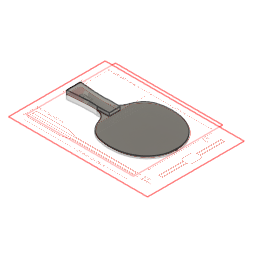
ping pong blade v3 (Autodesk Fusion 360 design; units mm, degrees)
Autodesk Fusion 360 part; units mm, degrees
sketch "Sketch1" plane through (0, 0, 0) normal (0, 0, 1) x (1, 0, 0)
  line L0 (-50.4364, 20) -> (-50.4364, 66.2164)
  line L1 (-50.4364, 20) -> (-50.4364, -26.2164)
  line L2 (-162.6012, 20) -> (-162.6012, 37.8)
  spline S0 degree 5 poles (-162.6012, 37.8) (-162.4087, 37.7675) (-161.9968, 37.7008) (-161.2988, 37.596) (-160.2074, 37.4467) (-158.5833, 37.2448) (-156.7226, 37.0291) (-154.6748, 36.8033) (-152.512, 36.5725) (-150.3117, 36.3424) (-148.1418, 36.1177) (-146.0475, 35.9017) (-144.0316, 35.6944) (-142.0557, 35.4931) (-140.0634, 35.2939) (-137.9994, 35.0931) (-135.8278, 34.8889) (-133.5564, 34.6833) (-131.2346, 34.4817) (-128.928, 34.291) (-126.6995, 34.1181) (-124.5892, 33.968) (-122.5913, 33.8422) (-120.6411, 33.7376) (-118.6447, 33.6482) (-116.5034, 33.5668) (-114.1389, 33.4868) (-111.5213, 33.4035) (-108.6885, 33.3162) (-105.7218, 33.2269) (-102.7286, 33.1405) (-99.8212, 33.0642) (-97.0976, 33.0075) (-94.623, 32.9812) (-92.4049, 32.998) (-90.397, 33.0706) (-88.525, 33.21) (-86.708, 33.4235) (-84.879, 33.7126) (-83.0115, 34.0709) (-81.1155, 34.4864) (-79.2188, 34.9473) (-77.3539, 35.4469) (-75.5416, 35.9885) (-73.7777, 36.5903) (-72.0452, 37.2766) (-70.3251, 38.0715) (-68.6068, 38.9915) (-66.9017, 40.0363) (-65.2418, 41.1906) (-63.6663, 42.433) (-62.2115, 43.7433) (-60.8996, 45.1106) (-59.7266, 46.542) (-58.6672, 48.0584) (-57.6848, 49.6888) (-56.7383, 51.464) (-55.792, 53.4107) (-54.8211, 55.5471) (-53.8091, 57.8853) (-52.7461, 60.4323) (-51.8509, 62.6395) (-51.1537, 64.3907) (-50.6774, 65.6008) (-50.4364, 66.2164) knots 0 0 0 0 0 0 0.01666667 0.03333333 0.05 0.06666667 0.08333333 0.1 0.11666667 0.13333333 0.15 0.16666667 0.18333333 0.2 0.21666667 0.23333333 0.25 0.26666667 0.28333333 0.3 0.31666667 0.33333333 0.35 0.36666667 0.38333333 0.4 0.41666667 0.43333333 0.45 0.46666667 0.48333333 0.5 0.51666667 0.53333333 0.55 0.56666667 0.58333333 0.6 0.61666667 0.63333333 0.65 0.66666667 0.68333333 0.7 0.71666667 0.73333333 0.75 0.76666667 0.78333333 0.8 0.81666667 0.83333333 0.85 0.86666667 0.88333333 0.9 0.91666667 0.93333333 0.95 0.96666667 0.98333333 1 1 1 1 1 1
  spline S1 degree 5 poles (-50.4364, 66.2164) (-50.3519, 66.4112) (-50.1757, 66.8083) (-49.8889, 67.4271) (-49.4619, 68.2982) (-48.8547, 69.4625) (-48.1772, 70.6978) (-47.4359, 71.9953) (-46.6416, 73.3403) (-45.8078, 74.7134) (-44.9479, 76.0937) (-44.072, 77.4613) (-43.185, 78.7999) (-42.2827, 80.0994) (-41.3532, 81.3565) (-40.382, 82.5722) (-39.3568, 83.7496) (-38.2715, 84.8926) (-37.1319, 86.0029) (-35.9566, 87.0799) (-34.7693, 88.121) (-33.5926, 89.1233) (-32.4408, 90.0841) (-31.3134, 91.0023) (-30.1901, 91.8786) (-29.0408, 92.7154) (-27.8344, 93.5153) (-26.5475, 94.2804) (-25.1741, 95.0118) (-23.7297, 95.7088) (-22.2422, 96.3696) (-20.7456, 96.9918) (-19.2732, 97.5726) (-17.8503, 98.1091) (-16.4878, 98.5993) (-15.1849, 99.042) (-13.9302, 99.4379) (-12.7036, 99.7901) (-11.4773, 100.1046) (-10.22, 100.3903) (-8.9052, 100.6573) (-7.5176, 100.9156) (-6.0613, 101.1732) (-4.5656, 101.4355) (-3.0718, 101.7048) (-1.6195, 101.9808) (-0.2335, 102.2603) (1.0906, 102.538) (2.3958, 102.806) (3.7421, 103.0559) (5.1885, 103.2799) (6.7748, 103.4722) (8.4989, 103.6309) (10.315, 103.7579) (12.155, 103.8571) (13.9436, 103.9335) (15.617, 103.9914) (17.138, 104.0331) (18.5172, 104.0573) (19.8025, 104.0605) (21.056, 104.0389) (22.3366, 103.9907) (23.6775, 103.9184) (25.0748, 103.8296) (26.5038, 103.7337) (27.9321, 103.6387) (29.332, 103.5492) (30.6963, 103.4618) (32.0362, 103.3676) (33.3674, 103.2568) (34.7009, 103.1228) (36.0308, 102.9669) (37.3268, 102.8014) (38.555, 102.6418) (39.6952, 102.5008) (40.7596, 102.3813) (41.8115, 102.2697) (42.9331, 102.1439) (44.1925, 101.9806) (45.6078, 101.7646) (47.1227, 101.4944) (48.6444, 101.1781) (50.0749, 100.8298) (51.3416, 100.4659) (52.4354, 100.1015) (53.4214, 99.7468) (54.3927, 99.4068) (55.4411, 99.0795) (56.6121, 98.7537) (57.9048, 98.4117) (59.2923, 98.0347) (60.7347, 97.6062) (62.1975, 97.1178) (63.6625, 96.5716) (65.1218, 95.9761) (66.575, 95.3435) (68.0244, 94.6863) (69.4712, 94.0139) (70.9122, 93.3296) (72.341, 92.6324) (73.7506, 91.9192) (75.1345, 91.1862) (76.489, 90.4307) (77.8147, 89.6534) (79.1164, 88.8568) (80.4014, 88.0438) (81.6783, 87.2155) (82.9563, 86.37) (84.2434, 85.4998) (85.546, 84.5942) (86.8673, 83.6418) (88.2065, 82.6336) (89.5581, 81.566) (90.91, 80.4435) (92.2446, 79.28) (93.5423, 78.0932) (94.7848, 76.902) (95.958, 75.7222) (97.0558, 74.5632) (98.0833, 73.4234) (99.0553, 72.2922) (99.9911, 71.1542) (100.9108, 69.9933) (101.8313, 68.7959) (102.7615, 67.5557) (103.7029, 66.273) (104.6516, 64.9514) (105.6008, 63.5956) (106.5423, 62.2091) (107.4689, 60.7914) (108.3755, 59.3369) (109.2582, 57.8381) (110.1142, 56.287) (110.941, 54.6779) (111.7362, 53.0089) (112.4967, 51.2846) (113.2191, 49.5157) (113.8998, 47.7159) (114.5354, 45.9004) (115.123, 44.083) (115.6604, 42.275) (116.1465, 40.4817) (116.5815, 38.702) (116.9663, 36.9306) (117.3026, 35.159) (117.5921, 33.377) (117.8368, 31.5747) (118.0382, 29.7435) (118.1974, 27.8777) (118.3152, 25.9734) (118.3921, 24.028) (118.4211, 22.4381) (118.4245, 21.2265) (118.4186, 20.4102) (118.4136, 20) knots 0 0 0 0 0 0 0.00666667 0.01333333 0.02 0.02666667 0.03333333 0.04 0.04666667 0.05333333 0.06 0.06666667 0.07333333 0.08 0.08666667 0.09333333 0.1 0.10666667 0.11333333 0.12 0.12666667 0.13333333 0.14 0.14666667 0.15333333 0.16 0.16666667 0.17333333 0.18 0.18666667 0.19333333 0.2 0.20666667 0.21333333 0.22 0.22666667 0.23333333 0.24 0.24666667 0.25333333 0.26 0.26666667 0.27333333 0.28 0.28666667 0.29333333 0.3 0.30666667 0.31333333 0.32 0.32666667 0.33333333 0.34 0.34666667 0.35333333 0.36 0.36666667 0.37333333 0.38 0.38666667 0.39333333 0.4 0.40666667 0.41333333 0.42 0.42666667 0.43333333 0.44 0.44666667 0.45333333 0.46 0.46666667 0.47333333 0.48 0.48666667 0.49333333 0.5 0.50666667 0.51333333 0.52 0.52666667 0.53333333 0.54 0.54666667 0.55333333 0.56 0.56666667 0.57333333 0.58 0.58666667 0.59333333 0.6 0.60666667 0.61333333 0.62 0.62666667 0.63333333 0.64 0.64666667 0.65333333 0.66 0.66666667 0.67333333 0.68 0.68666667 0.69333333 0.7 0.70666667 0.71333333 0.72 0.72666667 0.73333333 0.74 0.74666667 0.75333333 0.76 0.76666667 0.77333333 0.78 0.78666667 0.79333333 0.8 0.80666667 0.81333333 0.82 0.82666667 0.83333333 0.84 0.84666667 0.85333333 0.86 0.86666667 0.87333333 0.88 0.88666667 0.89333333 0.9 0.90666667 0.91333333 0.92 0.92666667 0.93333333 0.94 0.94666667 0.95333333 0.96 0.96666667 0.97333333 0.98 0.98666667 0.99333333 1 1 1 1 1 1
  line L3 (-50.4364, 18.5) -> (-162.6012, 18.5) construction
  line L4 (-50.4364, 18.5) -> (130, 18.5) construction
  spline S2 degree 5 poles (118.4136, 20) (118.4136, 19.94) (118.4136, 19.82) (118.4136, 19.64) (118.4136, 19.4) (118.4136, 19.1) (118.4136, 18.86) (118.4136, 18.68) (118.4136, 18.56) (118.4136, 18.5) knots 0 0 0 0 0 0 0.2 0.4 0.6 0.8 1 1 1 1 1 1
  line L5 (-162.6012, 18.5) -> (-162.6012, 20)
  spline S3 degree 5 poles (118.4136, 17) (118.4136, 17.06) (118.4136, 17.18) (118.4136, 17.36) (118.4136, 17.6) (118.4136, 17.9) (118.4136, 18.14) (118.4136, 18.32) (118.4136, 18.44) (118.4136, 18.5) knots 0 0 0 0 0 0 0.2 0.4 0.6 0.8 1 1 1 1 1 1
  line L6 (118.4136, 20.153) -> (118.4136, 19.847)
  line L7 (118.4136, 18.653) -> (118.4136, 18.347)
  line L8 (118.4136, 16.847) -> (118.4136, 17.153)
  line L9 (118.4136, 18.347) -> (118.4136, 18.653)
  spline S4 degree 5 poles (-162.6012, -0.8) (-162.4087, -0.7675) (-161.9968, -0.7008) (-161.2988, -0.596) (-160.2074, -0.4467) (-158.5833, -0.2448) (-156.7226, -0.0291) (-154.6748, 0.1967) (-152.512, 0.4275) (-150.3117, 0.6576) (-148.1418, 0.8823) (-146.0475, 1.0983) (-144.0316, 1.3056) (-142.0557, 1.5069) (-140.0634, 1.7061) (-137.9994, 1.9069) (-135.8278, 2.1111) (-133.5564, 2.3167) (-131.2346, 2.5183) (-128.928, 2.709) (-126.6995, 2.8819) (-124.5892, 3.032) (-122.5913, 3.1578) (-120.6411, 3.2624) (-118.6447, 3.3518) (-116.5034, 3.4332) (-114.1389, 3.5132) (-111.5213, 3.5965) (-108.6885, 3.6838) (-105.7218, 3.7731) (-102.7286, 3.8595) (-99.8212, 3.9358) (-97.0976, 3.9925) (-94.623, 4.0188) (-92.4049, 4.002) (-90.397, 3.9294) (-88.525, 3.79) (-86.708, 3.5765) (-84.879, 3.2874) (-83.0115, 2.9291) (-81.1155, 2.5136) (-79.2188, 2.0527) (-77.3539, 1.5531) (-75.5416, 1.0115) (-73.7777, 0.4097) (-72.0452, -0.2766) (-70.3251, -1.0715) (-68.6068, -1.9915) (-66.9017, -3.0363) (-65.2418, -4.1906) (-63.6663, -5.433) (-62.2115, -6.7433) (-60.8996, -8.1106) (-59.7266, -9.542) (-58.6672, -11.0584) (-57.6848, -12.6888) (-56.7383, -14.464) (-55.792, -16.4107) (-54.8211, -18.5471) (-53.8091, -20.8853) (-52.7461, -23.4323) (-51.8509, -25.6395) (-51.1537, -27.3907) (-50.6774, -28.6008) (-50.4364, -29.2164) knots 0 0 0 0 0 0 0.01666667 0.03333333 0.05 0.06666667 0.08333333 0.1 0.11666667 0.13333333 0.15 0.16666667 0.18333333 0.2 0.21666667 0.23333333 0.25 0.26666667 0.28333333 0.3 0.31666667 0.33333333 0.35 0.36666667 0.38333333 0.4 0.41666667 0.43333333 0.45 0.46666667 0.48333333 0.5 0.51666667 0.53333333 0.55 0.56666667 0.58333333 0.6 0.61666667 0.63333333 0.65 0.66666667 0.68333333 0.7 0.71666667 0.73333333 0.75 0.76666667 0.78333333 0.8 0.81666667 0.83333333 0.85 0.86666667 0.88333333 0.9 0.91666667 0.93333333 0.95 0.96666667 0.98333333 1 1 1 1 1 1
  line L10 (-171.3092, 39.2715) -> (-153.8933, 36.3285)
  line L11 (-56.351, 51.1084) -> (-44.5217, 81.3245)
  line L12 (-171.3092, -2.2715) -> (-153.8933, 0.6715)
  line L13 (-56.351, -14.1084) -> (-44.5217, -44.3245)
  spline S5 degree 5 poles (-50.4364, -29.2164) (-50.3519, -29.4112) (-50.1757, -29.8083) (-49.8889, -30.4271) (-49.4619, -31.2982) (-48.8547, -32.4625) (-48.1772, -33.6978) (-47.4359, -34.9953) (-46.6416, -36.3403) (-45.8078, -37.7134) (-44.9479, -39.0937) (-44.072, -40.4613) (-43.185, -41.7999) (-42.2827, -43.0994) (-41.3532, -44.3565) (-40.382, -45.5722) (-39.3568, -46.7496) (-38.2715, -47.8926) (-37.1319, -49.0029) (-35.9566, -50.0799) (-34.7693, -51.121) (-33.5926, -52.1233) (-32.4408, -53.0841) (-31.3134, -54.0023) (-30.1901, -54.8786) (-29.0408, -55.7154) (-27.8344, -56.5153) (-26.5475, -57.2804) (-25.1741, -58.0118) (-23.7297, -58.7088) (-22.2422, -59.3696) (-20.7456, -59.9918) (-19.2732, -60.5726) (-17.8503, -61.1091) (-16.4878, -61.5993) (-15.1849, -62.042) (-13.9302, -62.4379) (-12.7036, -62.7901) (-11.4773, -63.1046) (-10.22, -63.3903) (-8.9052, -63.6573) (-7.5176, -63.9156) (-6.0613, -64.1732) (-4.5656, -64.4355) (-3.0718, -64.7048) (-1.6195, -64.9808) (-0.2335, -65.2603) (1.0906, -65.538) (2.3958, -65.806) (3.7421, -66.0559) (5.1885, -66.2799) (6.7748, -66.4722) (8.4989, -66.6309) (10.315, -66.7579) (12.155, -66.8571) (13.9436, -66.9335) (15.617, -66.9914) (17.138, -67.0331) (18.5172, -67.0573) (19.8025, -67.0605) (21.056, -67.0389) (22.3366, -66.9907) (23.6775, -66.9184) (25.0748, -66.8296) (26.5038, -66.7337) (27.9321, -66.6387) (29.332, -66.5492) (30.6963, -66.4618) (32.0362, -66.3676) (33.3674, -66.2568) (34.7009, -66.1228) (36.0308, -65.9669) (37.3268, -65.8014) (38.555, -65.6418) (39.6952, -65.5008) (40.7596, -65.3813) (41.8115, -65.2697) (42.9331, -65.1439) (44.1925, -64.9806) (45.6078, -64.7646) (47.1227, -64.4944) (48.6444, -64.1781) (50.0749, -63.8298) (51.3416, -63.4659) (52.4354, -63.1015) (53.4214, -62.7468) (54.3927, -62.4068) (55.4411, -62.0795) (56.6121, -61.7537) (57.9048, -61.4117) (59.2923, -61.0347) (60.7347, -60.6062) (62.1975, -60.1178) (63.6625, -59.5716) (65.1218, -58.9761) (66.575, -58.3435) (68.0244, -57.6863) (69.4712, -57.0139) (70.9122, -56.3296) (72.341, -55.6324) (73.7506, -54.9192) (75.1345, -54.1862) (76.489, -53.4307) (77.8147, -52.6534) (79.1164, -51.8568) (80.4014, -51.0438) (81.6783, -50.2155) (82.9563, -49.37) (84.2434, -48.4998) (85.546, -47.5942) (86.8673, -46.6418) (88.2065, -45.6336) (89.5581, -44.566) (90.91, -43.4435) (92.2446, -42.28) (93.5423, -41.0932) (94.7848, -39.902) (95.958, -38.7222) (97.0558, -37.5632) (98.0833, -36.4234) (99.0553, -35.2922) (99.9911, -34.1542) (100.9108, -32.9933) (101.8313, -31.7959) (102.7615, -30.5557) (103.7029, -29.273) (104.6516, -27.9514) (105.6008, -26.5956) (106.5423, -25.2091) (107.4689, -23.7914) (108.3755, -22.3369) (109.2582, -20.8381) (110.1142, -19.287) (110.941, -17.6779) (111.7362, -16.0089) (112.4967, -14.2846) (113.2191, -12.5157) (113.8998, -10.7159) (114.5354, -8.9004) (115.123, -7.083) (115.6604, -5.275) (116.1465, -3.4817) (116.5815, -1.702) (116.9663, 0.0694) (117.3026, 1.841) (117.5921, 3.623) (117.8368, 5.4253) (118.0382, 7.2565) (118.1974, 9.1223) (118.3152, 11.0266) (118.3921, 12.972) (118.4211, 14.5619) (118.4245, 15.7735) (118.4186, 16.5898) (118.4136, 17) knots 0 0 0 0 0 0 0.00666667 0.01333333 0.02 0.02666667 0.03333333 0.04 0.04666667 0.05333333 0.06 0.06666667 0.07333333 0.08 0.08666667 0.09333333 0.1 0.10666667 0.11333333 0.12 0.12666667 0.13333333 0.14 0.14666667 0.15333333 0.16 0.16666667 0.17333333 0.18 0.18666667 0.19333333 0.2 0.20666667 0.21333333 0.22 0.22666667 0.23333333 0.24 0.24666667 0.25333333 0.26 0.26666667 0.27333333 0.28 0.28666667 0.29333333 0.3 0.30666667 0.31333333 0.32 0.32666667 0.33333333 0.34 0.34666667 0.35333333 0.36 0.36666667 0.37333333 0.38 0.38666667 0.39333333 0.4 0.40666667 0.41333333 0.42 0.42666667 0.43333333 0.44 0.44666667 0.45333333 0.46 0.46666667 0.47333333 0.48 0.48666667 0.49333333 0.5 0.50666667 0.51333333 0.52 0.52666667 0.53333333 0.54 0.54666667 0.55333333 0.56 0.56666667 0.57333333 0.58 0.58666667 0.59333333 0.6 0.60666667 0.61333333 0.62 0.62666667 0.63333333 0.64 0.64666667 0.65333333 0.66 0.66666667 0.67333333 0.68 0.68666667 0.69333333 0.7 0.70666667 0.71333333 0.72 0.72666667 0.73333333 0.74 0.74666667 0.75333333 0.76 0.76666667 0.77333333 0.78 0.78666667 0.79333333 0.8 0.80666667 0.81333333 0.82 0.82666667 0.83333333 0.84 0.84666667 0.85333333 0.86 0.86666667 0.87333333 0.88 0.88666667 0.89333333 0.9 0.90666667 0.91333333 0.92 0.92666667 0.93333333 0.94 0.94666667 0.95333333 0.96 0.96666667 0.97333333 0.98 0.98666667 0.99333333 1 1 1 1 1 1
  line L14 (-57.732, 49.3855) -> (-43.1407, 83.0474)
  line L15 (118.6965, 43.4057) -> (118.1307, -3.4057)
  line L16 (-57.732, -12.3855) -> (-43.1407, -46.0474)
  line L17 (118.6965, -6.4057) -> (118.1307, 40.4057)
  line L18 (-50.4364, 17) -> (-50.4364, -29.2164)
  line L19 (-162.6012, 18.5) -> (-162.6012, 17)
  line L20 (-162.6012, 17) -> (-162.6012, -0.8)
  line L21 (-50.4364, 18.5) -> (-162.6012, 18.5) construction
  line L22 (-50.4364, 17) -> (-50.4364, 63.2164)
  line L23 (-50.4364, 18.5) -> (130, 18.5) construction
  spline S6 degree 5 poles (-50.4364, 3.7923) (-50.7438, 3.7762) (-51.3916, 3.7437) (-52.4617, 3.6941) (-54.0888, 3.626) (-56.4744, 3.5374) (-59.2304, 3.4454) (-62.3595, 3.3497) (-65.8355, 3.2507) (-69.6225, 3.1487) (-73.6845, 3.0441) (-77.1311, 2.9586) (-79.8188, 2.8934) (-81.6556, 2.8495) (-82.5852, 2.8275) knots 0 0 0 0 0 0 0.1 0.2 0.3 0.4 0.5 0.6 0.7 0.8 0.9 1 1 1 1 1 1
  spline S7 degree 5 poles (-50.4364, 33.2077) (-50.7438, 33.2238) (-51.3916, 33.2563) (-52.4617, 33.3059) (-54.0888, 33.374) (-56.4744, 33.4626) (-59.2304, 33.5546) (-62.3595, 33.6503) (-65.8355, 33.7493) (-69.6225, 33.8513) (-73.6845, 33.9559) (-77.1311, 34.0414) (-79.8188, 34.1066) (-81.6556, 34.1505) (-82.5852, 34.1725) knots 0 0 0 0 0 0 0.1 0.2 0.3 0.4 0.5 0.6 0.7 0.8 0.9 1 1 1 1 1 1
  line L24 (-48.1326, 3.9128) -> (-52.7402, 3.6718)
  line L25 (-78.6222, 2.9214) -> (-86.5483, 2.7335)
  line L26 (-48.1326, 33.0872) -> (-52.7402, 33.3282)
  line L27 (-78.6222, 34.0786) -> (-86.5483, 34.2665)
  point P0 (-157.6424, 37.1373)
  point P1 (-147, 36)
  point P2 (-137, 35)
  point P3 (-125, 34)
  point P4 (-114.5, 33.5)
  point P5 (-96, 33)
  point P6 (-86.1097, 33.5281)
  point P7 (-77.5106, 35.4169)
  point P8 (-69.5576, 38.4987)
  point P9 (-62, 44)
  point P10 (-57, 51)
  point P11 (-48, 71)
  point P12 (-43.6519, 78.0886)
  point P13 (-38.6253, 84.5072)
  point P14 (-32.6321, 89.9204)
  point P15 (-27, 94)
  point P16 (-19.447, 97.499)
  point P17 (-13.2604, 99.6256)
  point P18 (-7.5765, 100.9016)
  point P19 (-0.462, 102.2162)
  point P20 (6.0339, 103.3762)
  point P21 (16, 104)
  point P22 (22, 104)
  point P23 (28.4178, 103.608)
  point P24 (34.5016, 103.1387)
  point P25 (39.708, 102.5023)
  point P26 (44, 102)
  point P27 (50.8727, 100.5933)
  point P28 (54.7775, 99.2918)
  point P29 (60.3888, 97.7009)
  point P30 (67.9381, 94.7217)
  point P31 (75.3742, 91.0457)
  point P32 (82, 87)
  point P33 (89, 82)
  point P34 (96.2547, 75.4003)
  point P35 (101.179, 69.6393)
  point P36 (106.1511, 62.7788)
  point P37 (111.2189, 54.0776)
  point P38 (115.4499, 42.962)
  point P39 (117.7448, 32.2051)
  point P40 (39.708, -65.5023)
  point P41 (-7.5765, -63.9016)
  point P42 (-62, -7)
  point P43 (-147, 1)
  point P44 (-38.6253, -47.5072)
  point P45 (-86.1097, 3.4719)
  point P46 (-125, 3)
  point P47 (-57, -14)
  point P48 (-77.5106, 1.5831)
  point P49 (-32.6321, -52.9204)
  point P50 (-48, -34)
  point P51 (106.1511, -25.7788)
  point P52 (60.3888, -60.7009)
  point P53 (-43.6519, -41.0886)
  point P54 (111.2189, -17.0776)
  point P55 (54.7775, -62.2918)
  point P56 (-137, 2)
  point P57 (-69.5576, -1.4987)
  point P58 (-27, -57)
  point P59 (44, -65)
  point P60 (89, -45)
  point P61 (16, -67)
  point P62 (-0.462, -65.2162)
  point P63 (-13.2604, -62.6256)
  point P64 (101.179, -32.6393)
  point P65 (-19.447, -60.499)
  point P66 (22, -67)
  point P67 (67.9381, -57.7217)
  point P68 (6.0339, -66.3762)
  point P69 (115.4499, -5.962)
  point P70 (117.7448, 4.7949)
  point P71 (34.5016, -66.1387)
  point P72 (28.4178, -66.608)
  point P73 (82, -50)
  point P74 (96.2547, -38.4003)
  point P75 (75.3742, -54.0457)
  point P76 (-114.5, 3.5)
  point P77 (50.8727, -63.5933)
  point P78 (-96, 4)
  point P79 (-157.6424, -0.1373)
  point P80 (-58.7708, 3.4622)
  point P81 (-58.7708, 33.5378)
  constraint equal L0 L1
  constraint coincident L4 S2.end
  constraint midpoint S1.end L6
  constraint midpoint S2.end L7
  constraint midpoint L2.end L10
  constraint midpoint L0.end L11
  constraint midpoint L0.end L14
  constraint midpoint S1.end L15
  constraint symmetric L0.start L4 L18.start
  constraint symmetric L2.start L4 L19.end
  constraint symmetric L0.end L4 S4.end
  constraint symmetric L1.end L4 L22.end
  constraint symmetric L2.end L4 S4.start
  constraint symmetric P0 L4 P79
  constraint symmetric P1 L4 P43
  constraint symmetric P2 L4 P56
  constraint symmetric P3 L4 P46
  constraint symmetric P4 L4 P76
  constraint symmetric P5 L4 P78
  constraint symmetric P6 L4 P45
  constraint symmetric P7 L4 P48
  constraint symmetric P8 L4 P57
  constraint symmetric P9 L4 P42
  constraint symmetric P10 L4 P47
  constraint symmetric P11 L4 P50
  constraint symmetric P12 L4 P53
  constraint symmetric P13 L4 P44
  constraint symmetric P14 L4 P49
  constraint symmetric P15 L4 P58
  constraint symmetric P16 L4 P65
  constraint symmetric P17 L4 P63
  constraint symmetric P18 L4 P41
  constraint symmetric P19 L4 P62
  constraint symmetric P20 L4 P68
  constraint symmetric P21 L4 P61
  constraint symmetric P22 L4 P66
  constraint symmetric P23 L4 P72
  constraint symmetric P24 L4 P71
  constraint symmetric P25 L4 P40
  constraint symmetric P26 L4 P59
  constraint symmetric P27 L4 P77
  constraint symmetric P28 L4 P55
  constraint symmetric P29 L4 P52
  constraint symmetric P30 L4 P67
  constraint symmetric P31 L4 P75
  constraint symmetric P32 L4 P73
  constraint symmetric P33 L4 P60
  constraint symmetric P34 L4 P74
  constraint symmetric P35 L4 P64
  constraint symmetric P36 L4 P51
  constraint symmetric P37 L4 P54
  constraint symmetric P38 L4 P69
  constraint symmetric P39 L4 P70
  constraint symmetric S1.end L4 S3.start
  constraint symmetric L3.start L4 L21.start
  constraint symmetric L3.end L4 L5.start
  constraint symmetric L23.end L4 L4.end
  constraint symmetric L4 S2.end S3.end
  constraint symmetric L4 L6.start L8.start
  constraint symmetric L4 L6.end L8.end
  constraint symmetric L4 L7.start L7.end
  constraint symmetric L4 L7.end L7.start
  constraint symmetric L4 L10.start L12.start
  constraint symmetric L4 L10.end L12.end
  constraint symmetric L4 L11.start L13.start
  constraint symmetric L4 L11.end L13.end
  constraint symmetric L4 L14.start L16.start
  constraint symmetric L4 L14.end L16.end
  constraint symmetric L4 L15.start L17.start
  constraint symmetric L4 L15.end L17.end
  constraint coincident L18 S6.start
  constraint coincident S4 S6.end
  constraint midpoint S6.start L24
  constraint midpoint S6.end L25
  constraint symmetric L3 S6.start S7.start
  constraint symmetric L3 P80 P81
  constraint symmetric L3 S6.end S7.end
  constraint symmetric L3 L24.start L26.start
  constraint symmetric L3 L24.end L26.end
  constraint symmetric L3 L25.start L27.start
  constraint symmetric L3 L25.end L27.end
extrude "Extrude1" add sketch "Sketch1" along normal mid plane 6 contours L0 L1 S1 S5 L15 L17 L18 L22 | L0 S0 L22 S7 L27 | L1 S4 L18 S6 L25 | S1 S2 L6 L15 L17 | S3 L8 S5 L15 L17 | S2 S3 L7 L9 L15 L17
extrude "Extrude2" add sketch "Sketch1" along normal mid plane 22 contours L0 L1 L2 S0 L5 S4 L18 L19 L20 L22 S6 S7 L25 L27
fillet "Fillet1" [rolled back] radius 6
chamfer "Chamfer1" [rolled back] distance 22 rotate angle 10
fillet "Fillet2" [rolled back] radius 4
